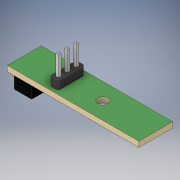
# Autodesk Inventor part: LineSensor
Saved by Autodesk Inventor 2019 (Build 230136000, 136)
## iProperties
Created: 2020-12-27
Part Number: LineSensor
Material: Типовые
Document SubType Name: Modeling
Designer: Professional
Density: 1 g/cm^3
Appearance: По умолчанию
Author: Professional
Autodesk Inventor part; units mm, degrees
ref_plane "YZ Plane" through (0, 0, 0) normal (1, 0, 0) x (0, 1, 0)
ref_plane "XZ Plane" through (0, 0, 0) normal (0, 1, 0) x (-1, 0, 0)
ref_plane "XY Plane" through (0, 0, 0) normal (0, 0, 1) x (1, 0, 0)
sketch "Эскиз2" plane through (0, 0, 0) normal (0, 1, 0) x (-1, 0, 0)
  line L0 (0, 0) -> (38.3359, 0) construction
  line L1 (38.3359, 0) -> (38.3359, -10) construction
  line L2 (38.3359, -10) -> (0, -10) construction
  line L3 (0, -10) -> (0, 0) construction
  line L4 (0, 0) -> (38.3359, 0)
  line L5 (38.3359, 0) -> (38.3359, -10)
  line L6 (38.3359, -10) -> (0, -10)
  line L7 (0, -10) -> (0, 0)
  circle A0 centre (15.6, -5) radius 1.5
  point P0 (0, -5)
  dimension "d1" = 10
  dimension "d11" = 15.6
  dimension "d12" = 3
  constraints: 8 end point, 2 horizontal, 2 parallel, 1 centre point, 1 horizontal alignment, 1 midpoint, 1 perpendicular, 2 other
  measures "d1" distance between parallel lines of L2 L0
  measures "d11" distance from line of L3 A0.centre
  measures "d12" diameter of A0
extrude "Выдавливание1" add sketch "Эскиз2" along normal blind 1.6
sketch "Эскиз3" plane through (0, 1.6, 0) normal (0, 1, 0) x (1, 0, 0)
  line L0 (0, 0) -> (-38.3359, 0) construction
  line L1 (-38.3359, 0) -> (-38.3359, 10) construction
  line L2 (-38.3359, 10) -> (0, 10) construction
  line L3 (0, 10) -> (0, 0) construction
  line L4 (-27.4359, 9) -> (-24.8359, 9)
  line L5 (-24.8359, 9) -> (-24.8359, 1)
  line L6 (-24.8359, 1) -> (-27.4359, 1)
  line L7 (-27.4359, 1) -> (-27.4359, 9)
  point P0 (-27.4359, 5)
  point P1 (-38.3359, 5)
  dimension "d43" = 2.6
  dimension "d50" = 8
  dimension "d51" = 10.9
  constraints: 8 end point, 2 coincident, 2 midpoint, 2 parallel, 1 horizontal, 1 horizontal alignment, 1 perpendicular, 2 other
  measures "d43" distance of L4.start L4.end
  measures "d50" distance between parallel lines of L4 L6
  measures "d51" distance between parallel lines of L1 L7
extrude "Выдавливание2" add sketch "Эскиз3" along normal blind 2.4
chamfer "Фаска1" distance 0.5 angle 45 4 edges at (-24.8359, 2.8, -1) (-27.4359, 2.8, -1) (-24.8359, 2.8, -9) (-27.4359, 2.8, -9)
sketch "Эскиз4" plane through (0, 4, 0) normal (0, 1, 0) x (1, 0, 0)
  line L0 (-26.5359, 8) -> (-25.7359, 8)
  line L1 (-25.7359, 8) -> (-25.7359, 7.2)
  line L2 (-25.7359, 7.2) -> (-26.5359, 7.2)
  line L3 (-26.5359, 7.2) -> (-26.5359, 8)
  line L4 (-26.5359, 5.4) -> (-25.7359, 5.4)
  line L5 (-25.7359, 5.4) -> (-25.7359, 4.6)
  line L6 (-25.7359, 4.6) -> (-26.5359, 4.6)
  line L7 (-26.5359, 4.6) -> (-26.5359, 5.4)
  line L8 (-26.5359, 2) -> (-25.7359, 2)
  line L9 (-25.7359, 2) -> (-25.7359, 2.8)
  line L10 (-25.7359, 2.8) -> (-26.5359, 2.8)
  line L11 (-26.5359, 2.8) -> (-26.5359, 2)
  line L12 (-27.4359, 8.5) -> (-26.9359, 9) projected
  line L13 (-27.4359, 8.5) -> (-27.4359, 1.5) projected
  line L14 (-26.9359, 1) -> (-27.4359, 1.5) projected
  line L15 (-26.9359, 1) -> (-25.3359, 1) projected
  line L16 (-24.8359, 1.5) -> (-25.3359, 1) projected
  line L17 (-24.8359, 1.5) -> (-24.8359, 8.5) projected
  line L18 (-25.3359, 9) -> (-24.8359, 8.5) projected
  line L19 (-25.3359, 9) -> (-26.9359, 9) projected
  line L20 (-27.4359, 5) -> (-24.8359, 5)
  point P0 (0, 0)
  point P1 (-26.5359, 5)
  point P2 (-26.1359, 5.4)
  point P3 (-26.1359, 9)
  dimension "d57" = 0.8
  dimension "d58" = 4.4
  constraints: 26 end point, 6 parallel, 5 midpoint, 4 point on line, 3 horizontal, 3 perpendicular, 2 equal length, 1 horizontal alignment, 1 vertical alignment, 2 other
  measures "d57" distance of L0.start L0.end
  measures "d58" distance between parallel lines of L10 L2
extrude "Выдавливание3" add sketch "Эскиз4" along normal blind 6 contours L0 L1 L2 L3 | L4 L5 L20 L7 | L20 L5 L6 L7 | L11 L10 L9 L8
chamfer "Фаска2" distance 0.2 angle 45 12 edges at (-26.1359, 10, -2) (-26.5359, 10, -2.4) (-26.1359, 10, -2.8) (-25.7359, 10, -2.4) (-26.1359, 10, -4.6) (-26.5359, 10, -5) (-26.1359, 10, -5.4) (-25.7359, 10, -5) (-26.1359, 10, -7.2) (-26.5359, 10, -7.6) (-26.1359, 10, -8) (-25.7359, 10, -7.6)
sketch "Эскиз5" plane through (0, 0, 0) normal (0, -1, 0) x (1, 0, 0)
  line L0 (-38.3359, -8.5) -> (-33.1359, -8.5)
  line L1 (-33.1359, -8.5) -> (-33.1359, -1.5)
  line L2 (-33.1359, -1.5) -> (-38.3359, -1.5)
  line L3 (-38.3359, -1.5) -> (-38.3359, -8.5)
  line L4 (-38.3359, 0) -> (-38.3359, -10) projected
  line L5 (0, -10) -> (-38.3359, -10) construction
  line L6 (-38.3359, -10) -> (-38.3359, 0) construction
  line L7 (-38.3359, 0) -> (0, 0) construction
  line L8 (0, 0) -> (0, -10) construction
  point P0 (0, 0)
  point P1 (-38.3359, -5)
  point P2 (-38.3359, -5)
  dimension "d106" = 5.2
  dimension "d109" = 7
  constraints: 8 end point, 2 coincident, 2 midpoint, 2 parallel, 1 horizontal, 1 perpendicular, 1 point on line, 2 other
  measures "d106" distance between parallel lines of L3 L1
  measures "d109" distance between parallel lines of L0 L2
sketch "Эскиз6" plane through (-38.3359, 0, -10) normal (-1, 0, 0) x (0, 0, 1)
  line L0 (10, 0) -> (0, 0) projected
  line L1 (10, 0) -> (10, 1.6) projected
  line L2 (0, 1.6) -> (10, 1.6) projected
  line L3 (0, 0) -> (0, 1.6) projected
  point P0 (10, 0)
extrude "Выдавливание4" add sketch "Эскиз6" along normal blind 0.5
extrude "Выдавливание5" add sketch "Эскиз5" along normal blind 5
